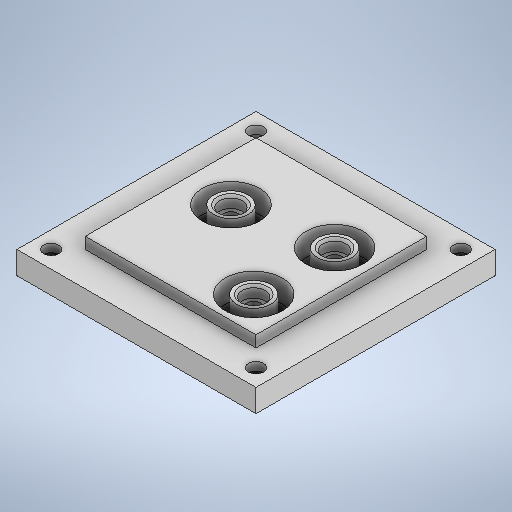
# Autodesk Inventor part: TS_Magazin_Grundplatte
Saved by Autodesk Inventor 2025.2 (Build 292293000, 293)
## iProperties
Created: 2025-06-01
Part Number: TS_Magazin_Grundplatte
Material: Generisch
Document SubType Name: Modeling
Designer: tino
Density: 1 g/cm^3
Appearance: Vorgabe
Author: tino
Autodesk Inventor part; units mm, degrees
ref_plane "YZ Plane" through (0, 0, 0) normal (1, 0, 0) x (0, 1, 0)
ref_plane "XZ Plane" through (0, 0, 0) normal (0, 1, 0) x (-1, 0, 0)
ref_plane "XY Plane" through (0, 0, 0) normal (0, 0, 1) x (1, 0, 0)
sketch "Skizze1" plane through (0, 0, 0) normal (0, 0, 1) x (1, 0, 0)
  line L0 (-52.5, 52.5) -> (52.5, 52.5)
  line L1 (52.5, 52.5) -> (52.5, -52.5)
  line L2 (52.5, -52.5) -> (-52.5, -52.5)
  line L3 (-52.5, -52.5) -> (-52.5, 52.5)
  line L4 (-52.5, 52.5) -> (52.5, -52.5) construction
  line L5 (52.5, 52.5) -> (-52.5, -52.5) construction
  point P0 (0, 0)
  dimension "d0" = 105
  dimension "d1" = 105
  constraints: 12 end point, 2 midpoint, 2 parallel, 1 horizontal, 1 perpendicular
  measures "d0" distance of L1.end L2.end
  measures "d1" distance of L0.end L1.end
extrude "Extrusion1" add sketch "Skizze1" along normal mid plane 15
sketch "Skizze2" plane through (0, 0, -7.5) normal (0, 0, -1) x (-1, 0, 0)
  point P0 (0, 0)
  point P1 (17.512, 6.5)
  point P2 (-21.618, -22.607)
  point P3 (-21.618, 12.918)
  dimension "d4" = 21.618
  dimension "d5" = 22.607
  dimension "d6" = 12.918
  dimension "d8" = 17.512
  dimension "d16" = 6.5
  constraints: 1 vertical alignment
  measures "d4" horizontal distance of point (-21.618, -22.607) point (0, 0)
  measures "d5" vertical distance of point (0, 0) point (-21.618, -22.607)
  measures "d6" vertical distance of point (-21.618, 12.918) point (0, 0)
  measures "d8" horizontal distance of point (0, 0) point (17.512, 6.5)
  measures "d16" vertical distance of point (0, 0) point (17.512, 6.5)
hole "Bohrung1" at (21.618, -22.607, -7.5) at (21.618, 12.918, -7.5) at (-17.512, 6.5, -7.5) direction (0, 0, 1) diameter 6.6 end through all counterbore diameter 11 counterbore depth 6.4
sketch "Skizze4" plane through (0, 0, 7.5) normal (0, 0, 1) x (1, 0, 0)
  circle A0 centre (-17.512, 6.5) radius 3.3 projected
  circle A1 centre (21.618, 12.918) radius 3.3 projected
  circle A2 centre (21.618, -22.607) radius 3.3 projected
  circle A3 centre (-17.512, 6.5) radius 5
  circle A4 centre (21.618, 12.918) radius 5
  circle A5 centre (21.618, -22.607) radius 5
  point P0 (0, 0)
  dimension "d24" = 10
  dimension "d25" = 10
  dimension "d26" = 10
  constraints: 3 centre point, 3 coincident
  measures "d24" diameter of A3
  measures "d25" diameter of A4
  measures "d26" diameter of A5
extrude "Extrusion2" cut sketch "Skizze4" against normal blind 5 contours A0 | A1 | A2 | A3 | A4 | A5
chamfer "Fasen1" distance 1 angle 45 3 edges at (-22.512, 6.5, 7.5) (16.618, 12.918, 7.5) (16.618, -22.607, 7.5)
sketch "Skizze5" plane through (0, 0, 7.5) normal (0, 0, 1) x (1, 0, 0)
  line L0 (-37.5, 37.5) -> (37.5, 37.5)
  line L1 (37.5, 37.5) -> (37.5, -37.5)
  line L2 (37.5, -37.5) -> (-37.5, -37.5)
  line L3 (-37.5, -37.5) -> (-37.5, 37.5)
  line L4 (-37.5, 37.5) -> (37.5, -37.5) construction
  line L5 (37.5, 37.5) -> (-37.5, -37.5) construction
  line L6 (52.5, 52.5) -> (-52.5, 52.5) projected
  line L7 (52.5, -52.5) -> (52.5, 52.5) projected
  line L8 (-52.5, 52.5) -> (-52.5, -52.5) projected
  line L9 (-52.5, -52.5) -> (52.5, -52.5) projected
  point P0 (0, 0)
  dimension "d32" = 15
  dimension "d33" = 15
  constraints: 12 end point, 2 midpoint, 2 parallel, 1 horizontal, 1 perpendicular
  measures "d32" distance between parallel lines of L0 L6
  measures "d33" distance between parallel lines of L7 L1
extrude "Extrusion3" cut sketch "Skizze5" against normal blind 5
sketch "Skizze6" plane through (0, 0, -7.5) normal (0, 0, -1) x (-1, 0, 0)
  line L0 (-52.5, -52.5) -> (52.5, -52.5) projected
  line L1 (52.5, -52.5) -> (52.5, 52.5) projected
  point P0 (0, 0)
  point P1 (45, -45)
  dimension "d36" = 7.5
  dimension "d37" = 7.5
  measures "d36" distance from line of point (45, -45) L0
  measures "d37" distance from line of L1 point (45, -45)
hole "Bohrung2" at (-45, -45, -7.5) direction (0, 0, 1) diameter 6.6 end through all counterbore diameter 11 counterbore depth 6.4
pattern_circular "Runde Anordnung1" count 4 over 360 about axis through (0, 0, -10) along (0, 0, 1) of "Bohrung2"
sketch "Skizze7" plane through (0, 0, 7.5) normal (0, 0, 1) x (1, 0, 0)
  circle A0 centre (-17.512, 6.5) radius 3.3 projected
  circle A1 centre (-17.512, 6.5) radius 7.5
  circle A2 centre (21.618, 12.918) radius 3.3 projected
  circle A3 centre (21.618, 12.918) radius 7.5
  circle A4 centre (21.618, -22.607) radius 3.3 projected
  circle A5 centre (21.618, -22.607) radius 7.5
  circle A6 centre (-17.512, 6.5) radius 12.5
  circle A7 centre (21.618, 12.918) radius 12.5
  circle A8 centre (21.618, -22.607) radius 5.5 projected
  circle A9 centre (21.618, -22.607) radius 12.5
  point P0 (0, 0)
  dimension "d48" = 15
  dimension "d49" = 15
  dimension "d50" = 15
  dimension "d51" = 25
  dimension "d52" = 25
  dimension "d53" = 25
  constraints: 6 centre point, 6 coincident
  measures "d48" diameter of A1
  measures "d49" diameter of A3
  measures "d50" diameter of A5
  measures "d51" diameter of A6
  measures "d52" diameter of A7
  measures "d53" diameter of A9
extrude "Extrusion4" cut sketch "Skizze7" against normal blind 10 contours A6 | A7 | A9
equation "\"d0\" = Breite_Magazin"
equation "\"d1\" = Tiefe_Magazin"
equation "\"d2\" = Hoehe_Bodenplatte"
equation "\"d27\" = Fuehrung_Tiefe"
equation "\"d29\" = Fase"
equation "\"d32\" = Wandstaerke"
equation "\"d33\" = Wandstaerke"
equation "\"d34\" = Fuehrung_Tiefe"
equation "\"d36\" = 0.5 * Wandstaerke"
equation "\"d37\" = 0.5 * Wandstaerke"
equation "\"d48\" = Feder_innen"
equation "\"d49\" = Feder_innen"
equation "\"d50\" = Feder_innen"
equation "\"d51\" = Feder_aussen"
equation "\"d52\" = Feder_aussen"
equation "\"d53\" = Feder_aussen"
equation "\"d54\" = Federfuehrung_Tiefe"
equation "\"Tiefe_Magazin\" = Breite_Magazin"
equation "\"Hoehe_Bodenplatte\" = 15"
equation "\"Fuehrung_Tiefe\" = 5"
equation "\"Fase\" = 1"
equation "\"Wandstaerke\" = 15"
equation "\"Feder_innen\" = 15"
equation "\"Feder_aussen\" = 25"
equation "\"Federfuehrung_Tiefe\" = 10"
equation "\"Breite_Magazin\" = 105"
